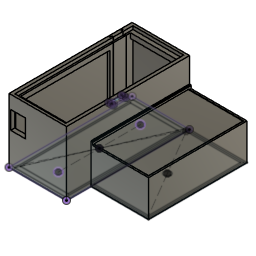
contolunit_casing v2 (Autodesk Fusion 360 design; units mm, degrees)
Autodesk Fusion 360 part; units mm, degrees
sketch "Sketch1" plane through (0, 0, 0) normal (0, 0, 1) x (1, 0, 0)
  line L0 (-17.5, 37.5) -> (17.5, 37.5)
  line L1 (17.5, 37.5) -> (17.5, -37.5)
  line L2 (17.5, -37.5) -> (-17.5, -37.5)
  line L3 (-17.5, -37.5) -> (-17.5, 37.5)
  line L4 (-14.5, 33.5) -> (14.5, 33.5)
  line L5 (14.5, 33.5) -> (14.5, -33.5)
  line L6 (14.5, -33.5) -> (-14.5, -33.5)
  line L7 (-14.5, -33.5) -> (-14.5, 33.5)
  line L8 (-15.5, 36) -> (15.5, 36)
  line L9 (15.5, 36) -> (15.5, -36)
  line L10 (15.5, -36) -> (-15.5, -36)
  line L11 (-15.5, -36) -> (-15.5, 36)
  line L12 (-14.5, -33.5) -> (14.5, 33.5) construction
  line L13 (-15.5, -36) -> (15.5, 36) construction
  line L14 (-17.5, -37.5) -> (17.5, 37.5) construction
  circle A0 centre (0, 25) radius 2
  circle A1 centre (0, -25) radius 2
  line L15 (0, 25) -> (0, 0) construction
  line L16 (0, -25) -> (0, 0) construction
  dimension "d1" = 35
  dimension "d2" = 75
  dimension "d3" = 29
  dimension "d4" = 67
  dimension "d5" = 31
  dimension "d6" = 72
  dimension "d7" = 4
  dimension "d8" = 4
  dimension "d9" = 25
  constraint horizontal L0
  constraint vertical L1
  constraint horizontal L2
  constraint vertical L3
  constraint horizontal L4
  constraint vertical L5
  constraint horizontal L6
  constraint vertical L7
  constraint horizontal L8
  constraint vertical L9
  constraint horizontal L10
  constraint vertical L11
  constraint midpoint L12 L15.end
  constraint midpoint L13 L15.end
  constraint midpoint L14 L15.end
  constraint coincident L15.end L16.end
  constraint coincident A0.centre L15.start
  constraint vertical L15
  constraint coincident A1.centre L16.start
  constraint parallel L15 L16
  constraint equal L15 L16
  measures "d1" distance of L0.start L0.end
  measures "d2" distance of L0.start L2.end
  measures "d3" distance of L4.start L4.end
  measures "d4" distance of L4.start L6.end
  measures "d5" distance of L8.start L8.end
  measures "d6" distance of L8.start L10.end
  measures "d7" diameter of A0
  measures "d8" diameter of A1
  measures "d9" distance of A0.centre L15.end
  measures "d62" distance of L6.end
extrude "Extrude1" add sketch "Sketch1" along normal blind 2 contours L4 L5 L6 L7 makes body 1
extrude "Extrude2" add sketch "Sketch1" along normal blind 37 contours L8 L9 L10 L11 bodies 1
extrude "Extrude3" add sketch "Sketch1" along normal blind 39 contours L0 L1 L2 L3 bodies 1
sketch "Sketch2" plane through (-17.5, 0, 0) normal (-1, 0, 0) x (0, -1, 0)
  line L0 (-37.5, 0) -> (37.5, 0)
  line L1 (37.5, 0) -> (37.5, 39)
  line L2 (37.5, 39) -> (-37.5, 39)
  line L3 (-37.5, 39) -> (-37.5, 0)
  line L4 (-30, 39) -> (-24, 39)
  line L5 (-24, 39) -> (-24, 4)
  line L6 (-24, 4) -> (-30, 4)
  line L7 (-30, 4) -> (-30, 39)
  dimension "d16" = 6
  dimension "d17" = 35
  constraint horizontal L4
  constraint vertical L5
  constraint horizontal L6
  constraint vertical L7
  constraint coincident L2 L4.start
  measures "d16" distance of L4.start L4.end
  measures "d17" distance of L4.start L6.end
extrude "Extrude4" cut sketch "Sketch2" against normal up to surface (3 mm away) contours L2 L4 L5 L6 L7 bodies 1
sketch "Sketch3" plane through (0, 0, 39) normal (0, 0, 1) x (-1, 0, 0)
  line L0 (17.5, -30) -> (15.5, -30)
  line L1 (15.5, -30) -> (15.5, -36)
  line L2 (15.5, -36) -> (-15.5, -36)
  line L3 (-15.5, -36) -> (-15.5, 36)
  line L4 (-15.5, 36) -> (15.5, 36)
  line L5 (15.5, 36) -> (15.5, -24)
  line L6 (15.5, -24) -> (17.5, -24)
  line L7 (17.5, -24) -> (17.5, 37.5)
  line L8 (17.5, 37.5) -> (-17.5, 37.5)
  line L9 (-17.5, 37.5) -> (-17.5, -37.5)
  line L10 (-17.5, -37.5) -> (17.5, -37.5)
  line L11 (17.5, -37.5) -> (17.5, -30)
  line L12 (15.5, -30) -> (14.5, -30)
  line L13 (14.5, -30) -> (14.5, -33.5)
  line L14 (14.5, -33.5) -> (-14.5, -33.5)
  line L15 (-14.5, -33.5) -> (-14.5, 33.5)
  line L16 (-14.5, 33.5) -> (14.5, 33.5)
  line L17 (14.5, 33.5) -> (14.5, -24)
  line L18 (14.5, -24) -> (15.5, -24)
  line L19 (15.5, -24) -> (15.5, 36)
  line L20 (15.5, 36) -> (-15.5, 36)
  line L21 (-15.5, 36) -> (-15.5, -36)
  line L22 (-15.5, -36) -> (15.5, -36)
  line L23 (15.5, -36) -> (15.5, -30)
  line L24 (17.5, -30) -> (14.5, -30)
  line L25 (14.5, -30) -> (14.5, -31)
  line L26 (14.5, -31) -> (17.5, -31)
  line L27 (17.5, -31) -> (17.5, -30)
  line L28 (17.5, -24) -> (14.5, -24)
  line L29 (14.5, -24) -> (14.5, -23)
  line L30 (14.5, -23) -> (17.5, -23)
  line L31 (17.5, -23) -> (17.5, -24)
  line L32 (16.5, -31) -> (16.5, -30)
  line L33 (16.5, -23) -> (16.5, -24)
  dimension "d20" = 3
  dimension "d21" = 1
  dimension "d22" = 3
  dimension "d23" = 1
  constraint horizontal L24
  constraint vertical L25
  constraint horizontal L26
  constraint vertical L27
  constraint coincident L0.start L11.end
  constraint horizontal L28
  constraint vertical L29
  constraint horizontal L30
  constraint vertical L31
  constraint coincident L6.end L7.start
  constraint coincident L26 L32.start
  constraint midpoint L0 L32.end
  constraint coincident L30 L33.start
  constraint midpoint L6 L33.end
  measures "d20" distance of L0.start L12.end
  measures "d21" distance of L0.start L26.end
  measures "d22" distance of L6.end L17.end
  measures "d23" distance of L6.end L30.end
extrude "Extrude5" cut sketch "Sketch3" against normal blind 35 contours L0 L11 L24 L26 L27 L32 | L1 L12 L13 L23 L24 L25 L26 | L6 L7 L28 L30 L31 L33 | L5 L17 L18 L19 L28 L29 L30 bodies 1
copy_body "Body->Comp1" bodies 1 removing the originals makes body 2 in component "base"
sketch "Sketch1 (2)" plane through (0, 0, 4) normal (0, 0, 1) x (-1, 0, 0) in component "protection"
  line L0 (14.5, -23) -> (14.5, -31)
  line L1 (14.5, -31) -> (15.5, -31)
  line L2 (15.5, -31) -> (15.5, -30)
  line L3 (15.5, -30) -> (16.5, -30)
  line L4 (16.5, -30) -> (16.5, -31)
  line L5 (16.5, -31) -> (17.5, -31)
  line L6 (17.5, -31) -> (17.5, -23)
  line L7 (17.5, -23) -> (16.5, -23)
  line L8 (16.5, -23) -> (16.5, -24)
  line L9 (16.5, -24) -> (15.5, -24)
  line L10 (15.5, -24) -> (15.5, -23)
  line L11 (15.5, -23) -> (14.5, -23)
  line L12 (16.6, -23.1) -> (16.6, -24.1)
  line L13 (16.6, -24.1) -> (15.4, -24.1)
  line L14 (15.4, -24.1) -> (15.4, -23.1)
  line L15 (15.4, -23.1) -> (14.6, -23.1)
  line L16 (14.6, -23.1) -> (14.6, -30.9)
  line L17 (14.6, -30.9) -> (15.4, -30.9)
  line L18 (15.4, -30.9) -> (15.4, -29.9)
  line L19 (15.4, -29.9) -> (16.6, -29.9)
  line L20 (16.6, -29.9) -> (16.6, -30.9)
  line L21 (16.6, -30.9) -> (17.4, -30.9)
  line L22 (17.4, -30.9) -> (17.4, -23.1)
  line L23 (17.4, -23.1) -> (16.6, -23.1)
  line L24 (14.6, -23.1) -> (14.5, -23.1)
  line L25 (17.4, -23.1) -> (17.5, -23.1)
  line L26 (14.6, -30.9) -> (14.5, -30.9)
  line L27 (17.4, -30.9) -> (17.5, -30.9)
  line L28 (16.5, -24.1) -> (16.5, -29.9)
  dimension "d26" = -0.1
  constraint coincident L0 L24.end
  constraint perpendicular L0 L24
  constraint coincident L6 L25.end
  constraint perpendicular L6 L25
  constraint coincident L0 L26.end
  constraint perpendicular L0 L26
  constraint coincident L6 L27.end
  constraint perpendicular L6 L27
  constraint coincident L13 L28.start
  constraint coincident L19 L28.end
  constraint perpendicular L19 L28
extrude "Extrude1'" add sketch "Sketch1 (2)" along normal blind 35 separate body contours L0 L16 L24 L26 | L13 L14 L15 L16 L17 L18 L19 L28 | L12 L13 L19 L20 L21 L22 L23 L28 | L6 L22 L25 L27 makes body 3 in component "protection"
sketch "Sketch2 (2)" plane through (0, 0, 39) normal (0, 0, 1) x (-1, 0, 0) in component "protection"
  line L0 (14.5, -30.9) -> (15.4, -30.9)
  line L1 (15.4, -30.9) -> (15.4, -29.9)
  line L2 (15.4, -29.9) -> (16.6, -29.9)
  line L3 (16.6, -29.9) -> (16.6, -30.9)
  line L4 (16.6, -30.9) -> (17.4, -30.9)
  line L5 (17.4, -30.9) -> (17.5, -30.9)
  line L6 (17.5, -30.9) -> (17.5, -23.1)
  line L7 (17.5, -23.1) -> (17.4, -23.1)
  line L8 (17.4, -23.1) -> (16.6, -23.1)
  line L9 (16.6, -23.1) -> (16.6, -24.1)
  line L10 (16.6, -24.1) -> (15.4, -24.1)
  line L11 (15.4, -24.1) -> (15.4, -23.1)
  line L12 (15.4, -23.1) -> (14.5, -23.1)
  line L13 (14.5, -23.1) -> (14.5, -30.9)
  line L14 (15.5, -29.9) -> (15.5, -24.1)
  constraint coincident L2 L14.start
  constraint coincident L10 L14.end
  constraint perpendicular L10 L14
extrude "Extrude4'" cut sketch "Sketch2 (2)" against normal blind 2 contours L0 L1 L2 L10 L11 L12 L13 L14 bodies 3 in component "protection"
sketch "Sketch4" plane through (0, 0, 2) normal (0, 0, 1) x (-1, 0, 0)
  circle A0 centre (0, -25) radius 2
  circle A1 centre (0, 25) radius 2
  line L0 (14.5, 33.5) -> (-14.5, 33.5)
  line L1 (-14.5, 33.5) -> (-14.5, -33.5)
  line L2 (-14.5, -33.5) -> (14.5, -33.5)
  line L3 (14.5, -33.5) -> (14.5, 33.5)
  line L4 (17.5, -37.5) -> (17.5, 37.5)
  line L5 (17.5, 37.5) -> (-17.5, 37.5)
  line L6 (-17.5, 37.5) -> (-17.5, -37.5)
  line L7 (-17.5, -37.5) -> (17.5, -37.5)
  line L8 (-14.5, -33.5) -> (-14.5, 33.5)
  line L9 (-14.5, 33.5) -> (14.5, 33.5)
  line L10 (14.5, 33.5) -> (14.5, -33.5)
  line L11 (14.5, -33.5) -> (-14.5, -33.5)
  circle A2 centre (0, 25) radius 2
  circle A3 centre (0, -25) radius 2
  line L12 (-16, -35) -> (16, -35)
  line L13 (16, -35) -> (16, 35)
  line L14 (16, 35) -> (-16, 35)
  line L15 (-16, 35) -> (-16, -35)
  line L16 (16, -35) -> (14.5, -35)
  line L17 (14.5, -35) -> (14.5, -20.9735)
  line L18 (14.5, -20.9735) -> (16, -20.9735)
  line L19 (16, -20.9735) -> (16, -35)
  dimension "d39" = 1.5
  constraint horizontal L16
  constraint vertical L17
  constraint horizontal L18
  constraint vertical L19
  constraint coincident L10 L17.end
extrude "Extrude1''" cut sketch "Sketch4" along normal blind 32 contours L0 L1 L2 L3 L8 L9 L10 L11 L12 L13 L14 L15 L17 L18 bodies 2 in component "base"
chamfer "Chamfer1" distance 1.5 angle 45 4 edges at (-16, -7.0132, 34) (0, -35, 34) (0.75, 35, 34) (16, 0, 34) on bodies 2 in component "base"
sketch "Sketch5" plane through (0, 0, 0) normal (0, 0, 1) x (1, 0, 0)
  line L0 (-17.5, -37.5) -> (-17.5, 37.5)
  line L1 (-17.5, 37.5) -> (17.5, 37.5)
  line L2 (17.5, 37.5) -> (17.5, -37.5)
  line L3 (17.5, -37.5) -> (-17.5, -37.5)
  circle A0 centre (0, -25) radius 2
  circle A1 centre (0, 25) radius 2
  line L4 (17.5, 37.5) -> (52.5, 37.5)
  line L5 (52.5, 37.5) -> (52.5, -22.5)
  line L6 (52.5, -22.5) -> (17.5, -22.5)
  line L7 (17.5, -22.5) -> (17.5, 37.5)
  line L8 (17.5, 35.5) -> (50.5, 35.5)
  line L9 (50.5, 35.5) -> (50.5, -20.5)
  line L10 (50.5, -20.5) -> (17.5, -20.5)
  line L11 (17.5, -20.5) -> (17.5, 35.5)
  line L12 (51.5, -21.5) -> (16.5, -21.5)
  line L13 (16.5, -21.5) -> (16.5, 36.5)
  line L14 (16.5, 36.5) -> (51.5, 36.5)
  line L15 (51.5, 36.5) -> (51.5, -21.5)
  line L16 (17.5, 35.5) -> (50.5, -20.5) construction
  circle A2 centre (34, 7.5) radius 2
  point P0 (34, 7.5)
  dimension "d43" = 35
  dimension "d44" = 60
  dimension "d45" = 2
  dimension "d46" = 2
  dimension "d47" = 2
  dimension "d48" = -1
  dimension "d49" = 4
  constraint horizontal L4
  constraint vertical L5
  constraint horizontal L6
  constraint vertical L7
  constraint coincident L1.end L2.start
  constraint horizontal L8
  constraint vertical L9
  constraint horizontal L10
  constraint vertical L11
  constraint coincident L2 L8.start
  constraint midpoint L16 P0
  constraint coincident P0 A2.centre
  measures "d43" distance of L1.end L4.end
  measures "d44" distance of L1.end L6.end
  measures "d45" distance of L6 L10
  measures "d46" distance of L4 L8
  measures "d47" distance of L5 L9
  measures "d49" diameter of A2
extrude "Extrude2'" add sketch "Sketch5" along normal blind 1.5 contours L2 L7 L8 L9 L10 L11 bodies 2 in component "base"
sketch "Sketch1 (3)" plane through (17.5, 0, 0) normal (1, 0, 0) x (0, 1, 0) in component "base"
  line L0 (-20.5, 0) -> (-20.5, 1.5)
  line L1 (-20.5, 1.5) -> (35.5, 1.5)
  line L2 (35.5, 1.5) -> (35.5, 0)
  line L3 (35.5, 0) -> (37.5, 0)
  line L4 (37.5, 0) -> (37.5, 39)
  line L5 (37.5, 39) -> (-37.5, 39)
  line L6 (-37.5, 39) -> (-37.5, 0)
  line L7 (-37.5, 0) -> (-20.5, 0)
  line L8 (33.5, 1.5) -> (3.5, 1.5)
  line L9 (3.5, 1.5) -> (3.5, 13.5)
  line L10 (3.5, 13.5) -> (33.5, 13.5)
  line L11 (33.5, 13.5) -> (33.5, 1.5)
  dimension "d52" = 30
  dimension "d53" = 12
  dimension "d54" = 2
  constraint horizontal L8
  constraint vertical L9
  constraint horizontal L10
  constraint vertical L11
  constraint coincident L1 L8.start
  measures "d52" distance of L8.start L8.end
  measures "d53" distance of L8.start L10.end
  measures "d54" distance of L1.end L8.start
extrude "Extrude3'" cut sketch "Sketch1 (3)" against normal up to surface (1.5 mm away) contours L1 L8 L9 L10 L11 bodies 2 in component "base"
extrude "Extrude4''" add sketch "Sketch5" along normal blind 20 contours L2 L7 L8 L9 L10 L12 L14 L15 bodies 2 in component "base"
extrude "Extrude5'" add sketch "Sketch5" along normal blind 22 contours L2 L4 L5 L6 L7 L12 L14 L15 bodies 2 in component "base"
chamfer "Chamfer2" distance 4 angle 45 4 edges at (17.5, -20.5, 10.75) (50.5, -20.5, 10.75) (50.5, 35.5, 10.75) (17.5, 35.5, 10.75) on bodies 2 in component "base"
sketch "Sketch2 (3)" plane through (17.5, 0, 0) normal (1, 0, 0) x (0, 1, 0) in component "base"
  line L0 (31.5, 13.5) -> (31.5, 20)
  line L1 (31.5, 20) -> (36.5, 20)
  line L2 (36.5, 20) -> (36.5, 22)
  line L3 (36.5, 22) -> (37.5, 22)
  line L4 (37.5, 22) -> (37.5, 39)
  line L5 (37.5, 39) -> (-37.5, 39)
  line L6 (-37.5, 39) -> (-37.5, 0)
  line L7 (-37.5, 0) -> (-22.5, 0)
  line L8 (-22.5, 0) -> (-22.5, 22)
  line L9 (-22.5, 22) -> (-21.5, 22)
  line L10 (-21.5, 22) -> (-21.5, 20)
  line L11 (-21.5, 20) -> (-16.5, 20)
  line L12 (-16.5, 20) -> (-16.5, 1.5)
  line L13 (-16.5, 1.5) -> (3.5, 1.5)
  line L14 (3.5, 1.5) -> (3.5, 13.5)
  line L15 (3.5, 13.5) -> (31.5, 13.5)
  line L16 (-22.5, 22) -> (37.5, 22)
  line L17 (37.5, 22) -> (37.5, 24)
  line L18 (37.5, 24) -> (-22.5, 24)
  line L19 (-22.5, 24) -> (-22.5, 22)
  dimension "d62" = 2
  constraint horizontal L16
  constraint vertical L17
  constraint horizontal L18
  constraint vertical L19
  constraint coincident L8.end L9.start
  measures "d62" distance of L8.end L18.end
extrude "Extrude6" add sketch "Sketch2 (3)" along normal blind 1 contours L3 L4 L9 L16 L17 L18 L19 bodies 2 in component "base"
chamfer "Chamfer3" distance 0.5 angle 45 1 edges at (18.5, 7.5, 22) on bodies 2 in component "base"
chamfer "Chamfer4" distance 0.3 angle 45 1 edges at (18.5, 7.5, 24) on bodies 2 in component "base"
sketch "Sketch1 (4)" plane through (0, 0, 20) normal (0, 0, 1) x (-1, 0, 0) in component "lid"
  line L0 (-21.5, -35.5) -> (-46.5, -35.5)
  line L1 (-46.5, -35.5) -> (-50.5, -31.5)
  line L2 (-50.5, -31.5) -> (-50.5, 16.5)
  line L3 (-50.5, 16.5) -> (-46.5, 20.5)
  line L4 (-46.5, 20.5) -> (-21.5, 20.5)
  line L5 (-21.5, 20.5) -> (-17.5, 16.5)
  line L6 (-17.5, 16.5) -> (-17.5, 21.5)
  line L7 (-17.5, 21.5) -> (-51.5, 21.5)
  line L8 (-51.5, 21.5) -> (-51.5, -36.5)
  line L9 (-51.5, -36.5) -> (-17.5, -36.5)
  line L10 (-17.5, -36.5) -> (-17.5, -31.5)
  line L11 (-17.5, -31.5) -> (-21.5, -35.5)
  line L12 (-46.5, -35.5) -> (-50.5, -31.5)
  line L13 (-50.5, -31.5) -> (-50.5, 16.5)
  line L14 (-50.5, 16.5) -> (-46.5, 20.5)
  line L15 (-46.5, 20.5) -> (-21.5, 20.5)
  line L16 (-21.5, 20.5) -> (-17.5, 16.5)
  line L17 (-17.5, 21.5) -> (-17.5, 16.5)
  line L18 (-51.5, 21.5) -> (-17.5, 21.5)
  line L19 (-51.5, -36.5) -> (-51.5, 21.5)
  line L20 (-17.5, -36.5) -> (-51.5, -36.5)
  line L21 (-17.5, -31.5) -> (-17.5, -36.5)
  line L22 (-17.5, -31.5) -> (-21.5, -35.5)
  line L23 (-21.5, -35.5) -> (-46.5, -35.5)
  line L24 (-17.5, 16.5) -> (-17.5, -31.5)
  line L25 (14.5, -23) -> (15.5, -23)
  line L26 (15.5, -23) -> (15.5, -24)
  line L27 (15.5, -24) -> (16.5, -24)
  line L28 (16.5, -24) -> (16.5, -23)
  line L29 (16.5, -23) -> (17.5, -23)
  line L30 (17.5, -23) -> (17.5, 37.5)
  line L31 (17.5, 37.5) -> (-17.5, 37.5)
  line L32 (-17.5, 37.5) -> (-17.5, 22.5)
  line L33 (-17.5, 22.5) -> (-52.5, 22.5)
  line L34 (-52.5, 22.5) -> (-52.5, -37.5)
  line L35 (-52.5, -37.5) -> (17.5, -37.5)
  line L36 (17.5, -37.5) -> (17.5, -31)
  line L37 (17.5, -31) -> (16.5, -31)
  line L38 (16.5, -31) -> (16.5, -30)
  line L39 (16.5, -30) -> (15.5, -30)
  line L40 (15.5, -30) -> (15.5, -31)
  line L41 (15.5, -31) -> (14.5, -31)
  line L42 (14.5, -31) -> (14.5, -35)
  line L43 (14.5, -35) -> (-16, -35)
  line L44 (-16, -35) -> (-16, 35)
  line L45 (-16, 35) -> (16, 35)
  line L46 (16, 35) -> (16, -20.9735)
  line L47 (16, -20.9735) -> (14.5, -20.9735)
  line L48 (14.5, -20.9735) -> (14.5, -23)
  line L49 (-17.7, 16.5) -> (-17.7, -31.5)
  line L50 (-17.7, -31.5) -> (-17.7, -36.3)
  line L51 (-17.7, -36.3) -> (-51.3, -36.3)
  line L52 (-51.3, -36.3) -> (-51.3, 21.3)
  line L53 (-51.3, 21.3) -> (-17.7, 21.3)
  line L54 (-17.7, 21.3) -> (-17.7, 16.5)
  dimension "d67" = 0.2
extrude "Extrude1'''" add sketch "Sketch1 (4)" along normal blind 1.9 separate body contours L0 L1 L2 L3 L4 L5 L11 L12 L13 L14 L15 L16 L22 L23 L50 L51 L52 L53 L54 | L0 L1 L2 L3 L4 L5 L11 L12 L13 L14 L15 L16 L22 L23 L49 L50 L54 makes body 4 in component "lid"
sketch "Sketch3 (2)" plane through (50.5, 0, 0) normal (-1, 0, 0) x (0, -1, 0) in component "base"
  line L0 (-31.5, 20) -> (-31.5, 1.5)
  line L1 (-31.5, 1.5) -> (16.5, 1.5)
  line L2 (16.5, 1.5) -> (16.5, 20)
  line L3 (16.5, 20) -> (-31.5, 20)
  line L4 (-7.5, 20) -> (-7.5, 1.5) construction
  line L5 (-9.5, 20) -> (-5.5, 20)
  line L6 (-5.5, 20) -> (-5.5, 1.5)
  line L7 (-5.5, 1.5) -> (-9.5, 1.5)
  line L8 (-9.5, 1.5) -> (-9.5, 20)
  dimension "d70" = 4
  constraint midpoint L3 L4.start
  constraint midpoint L1 L4.end
  constraint horizontal L5
  constraint vertical L6
  constraint horizontal L7
  constraint vertical L8
  constraint coincident L1 L6.end
  constraint coincident L3 L5.start
  constraint midpoint L4.start L5
  measures "d70" distance of L5.start L5.end
extrude "Extrude7" add sketch "Sketch3 (2)" along normal blind 3 contours L1 L3 L5 L6 L7 L8 bodies 2 in component "base"
chamfer "Chamfer5" distance 1.3 angle 45 4 edges at (50.5, 5.5, 10.75) (50.5, 9.5, 10.75) (47.5, 9.5, 10.75) (47.5, 5.5, 10.75) on bodies 2 in component "base"
sketch "Sketch4 (2)" plane through (0, -37.5, 0) normal (0, -1, 0) x (1, 0, 0) in component "base"
  line L0 (-17.5, 0) -> (17.5, 0)
  line L1 (17.5, 0) -> (17.5, 39)
  line L2 (17.5, 39) -> (-17.5, 39)
  line L3 (-17.5, 39) -> (-17.5, 0)
  line L4 (15.5, 37) -> (-15.5, 37)
  line L5 (-15.5, 37) -> (-15.5, 39)
  line L6 (-15.5, 39) -> (15.5, 39)
  line L7 (15.5, 39) -> (15.5, 37)
  line L8 (-15.5, 37) -> (-15.5, 0) construction
  line L9 (-16.5, 31) -> (-7.5, 31)
  line L10 (-7.5, 31) -> (-7.5, 20)
  line L11 (-7.5, 20) -> (-16.5, 20)
  line L12 (-16.5, 20) -> (-16.5, 31)
  dimension "d74" = 1
  dimension "d75" = 9
  dimension "d76" = 11
  dimension "d77" = 6
  constraint coincident L4.end L5.start
  constraint coincident L0 L8.end
  constraint perpendicular L0 L8
  constraint horizontal L9
  constraint vertical L10
  constraint horizontal L11
  constraint vertical L12
  measures "d74" distance of L8 L12
  measures "d75" distance of L10 L12
  measures "d76" distance of L9 L11
  measures "d77" distance of L4 L9
extrude "Extrude8" cut sketch "Sketch4 (2)" against normal up to surface (2.5 mm away) contours L9 L10 L11 L12 bodies 2 in component "base"
component "base" placed x (1, 0, 0) y (0, 1, 0) z (0, 0, 1) at (0, 0, 0)
component "protection" placed x (1, 0, 0) y (0, 1, 0) z (0, 0, 1) at (0, 0, 0)
component "lid" placed x (1, 0, 0) y (0, 1, 0) z (0, 0, 1) at (0, 0, 0)
